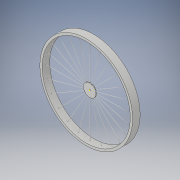
# Autodesk Inventor part: 輪子
Saved by Autodesk Inventor 2019 (Build 230136000, 136)
## iProperties
Created: 2021-03-29
Part Number: 輪子
Material: 一般
Document SubType Name: Modeling
Designer: cadlab
Density: 1 g/cm^3
Appearance: 預設
Author: cadlab
Autodesk Inventor part; units mm, degrees
ref_plane "YZ Plane" through (0, 0, 0) normal (1, 0, 0) x (0, 1, 0)
ref_plane "XZ Plane" through (0, 0, 0) normal (0, 1, 0) x (-1, 0, 0)
ref_plane "XY Plane" through (0, 0, 0) normal (0, 0, 1) x (1, 0, 0)
sketch "草圖1" plane through (0, 0, 0) normal (0, 0, 1) x (1, 0, 0)
  circle A0 centre (0, 0) radius 368
  circle A1 centre (0, 0) radius 350
  line L0 (30, 0) -> (350, 0)
  dimension "d4" = 700
  dimension "d0" = 736
  constraints: 2 end point, 1 centre point, 1 coincident, 1 horizontal, 1 horizontal alignment, 2 other
  measures "d0" diameter of A0
ref_plane "工作平面1" through (350, 0, 0) normal (1, 0, 0) x (0, 1, 0)
extrude "擠出2" add sketch "草圖1" along normal mid plane 60
sketch "草圖4" plane through (0, 0, 0) normal (0, 0, 1) x (1, 0, 0)
  circle A0 centre (0, 0) radius 50
  circle A1 centre (0, 0) radius 5
  dimension "d11" = 100
  dimension "d12" = 10
  constraints: 2 centre point, 2 coincident
  measures "d11" diameter of A0
  measures "d12" diameter of A1
extrude "擠出3" add sketch "草圖4" along normal mid plane 5
sketch "草圖5" plane through (0, 0, 2.5) normal (0, 0, 1) x (1, 0, 0)
  point P0 (0, 0)
sketch "草圖6" plane through (0, 0, 0) normal (0, 0, 1) x (1, 0, 0)
  circle A0 centre (0, 0) radius 50 projected
  line L0 (50, 0) -> (350, 0)
  circle A1 centre (0, 0) radius 350 projected
  constraints: 2 end point, 2 horizontal alignment, 1 horizontal, 2 other
ref_plane "工作平面2" through (350, 0, 0) normal (1, 0, 0) x (0, 1, 0)
sketch "草圖7" plane through (350, 0, 0) normal (1, 0, 0) x (0, 1, 0)
  line L0 (-50, -2.5) -> (50, -2.5) projected
  circle A0 centre (0, 0) radius 1.5
  dimension "d16" = 3
  constraints: 1 centre point, 1 coincident
  measures "d16" diameter of A0
sweep "掃掠2" add profiles "草圖7" path "草圖6" path curves L0
pattern_circular "環形陣列1" count 24 over 360 about axis through (0, 0, 0) along (0, 0, 1)
